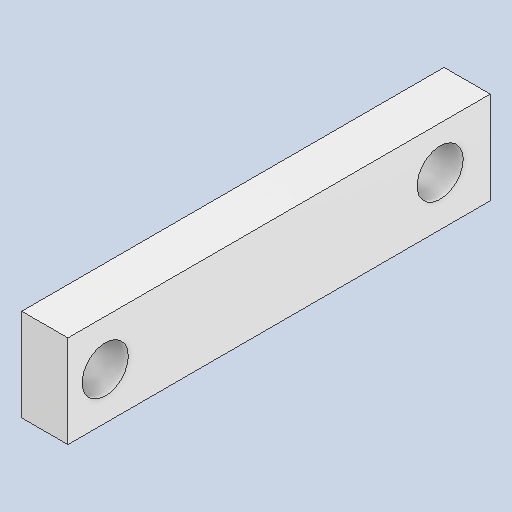
# Autodesk Inventor part: expo arm
Saved by Autodesk Inventor 2023 (Build 270158000, 158)
## iProperties
Created: 2022-06-23
Part Number: expo arm
Material: PVC, Unplasticized
Document SubType Name: Modeling
Designer: Shreyas P Mutnal
Density: 1.29 g/cm^3
Appearance: Smooth - White
Author: Shreyas P Mutnal
Autodesk Inventor part; units mm, degrees
ref_plane "YZ Plane" through (0, 0, 0) normal (1, 0, 0) x (0, 1, 0)
ref_plane "XZ Plane" through (0, 0, 0) normal (0, 1, 0) x (-1, 0, 0)
ref_plane "XY Plane" through (0, 0, 0) normal (0, 0, 1) x (1, 0, 0)
sketch "Sketch1" plane through (0, 0, 0) normal (1, 0, 0) x (0, 1, 0)
  line L0 (14.3117, 38.8012) -> (-5.6883, 38.8012)
  line L1 (-5.6883, 38.8012) -> (-5.6883, -52.6055)
  line L2 (-5.6883, -52.6055) -> (14.3117, -52.6055)
  line L3 (14.3117, -52.6055) -> (14.3117, 38.8012)
  point P0 (0, 0)
  dimension "d1" = 20
  constraints: 8 end point, 2 parallel, 1 horizontal, 1 perpendicular
  measures "d1" distance of L2.end L1.end
extrude "Extrusion1" add sketch "Sketch1" along normal blind 10
sketch "Sketch2" plane through (0, 0, 0) normal (-1, 0, 0) x (0, 0, 1)
  point P0 (0, 0)
  point P1 (30.7387, 4.3762)
hole "Hole1" at (0, 4.3762, 30.7387) direction (1, 0, 0) diameter 10 end through all
sketch "Sketch3" plane through (0, 0, 0) normal (-1, 0, 0) x (0, 0, 1)
  point P0 (0, 0)
  point P1 (-41.7535, 5.0249)
hole "Hole2" at (0, 5.0249, -41.7535) direction (1, 0, 0) diameter 10 end through all
body "Solid1"
